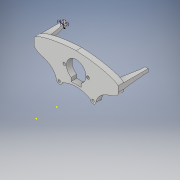
# Autodesk Inventor part: turret_base
Saved by Autodesk Inventor 2019 (Build 230136000, 136)
## iProperties
Created: 2019-04-21
Part Number: turret_base
Material: Ogólny
Document SubType Name: Modeling
Designer: terg
Density: 1 g/cm^3
Appearance: Domyślna
Author: terg
Autodesk Inventor part; units mm, degrees
ref_plane "XZ Plane" through (0, 0, 0) normal (0, 1, 0) x (-1, 0, 0)
sketch "Szkic2" plane through (0, 0, 0) normal (0, 0, 1) x (1, 0, 0)
  line L0 (4.75, 102.75) -> (9.25, 102.75)
  line L1 (9.25, 102.75) -> (9.25, 107.25)
  line L2 (9.25, 107.25) -> (4.75, 107.25)
  line L3 (4.75, 107.25) -> (4.75, 102.75)
  line L4 (4.75, 102.75) -> (9.25, 107.25) construction
  line L5 (9.25, 102.75) -> (4.75, 107.25) construction
  point P0 (0, 0)
  point P1 (64.95, 71.5)
  point P2 (7, 105)
  dimension "d1" = 4.5
  dimension "d2" = 4.5
  constraints: 12 end point, 2 midpoint, 2 parallel, 1 horizontal, 1 perpendicular, 1 other
  measures "d1" distance of L2.end L1.end
  measures "d2" distance of L1.end L0.end
ref_plane "Płaszczyzna konstrukcyjna1" through (64.95, 71.5, 0) normal (1, 0, 0) x (0, 1, 0)
ref_plane "Płaszczyzna konstrukcyjna2" through (0, 0, 29) normal (0, 0, 1) x (1, 0, 0)
sketch "Szkic3" plane through (0, 0, 29) normal (0, 0, 1) x (1, 0, 0)
  circle A0 centre (40.75, 71) radius 1.75 projected
  point P0 (0, 0)
extrude "Wyciągnięcie proste1" add sketch "Szkic2" against normal blind 6
sketch "Szkic4" plane through (0, 0, 0) normal (0, 0, 1) x (1, 0, 0)
  line L0 (4.75, 102.75) -> (9.25, 102.75) projected
  line L1 (9.25, 102.75) -> (9.25, 107.25) projected
  line L2 (9.25, 107.25) -> (4.75, 107.25) projected
  line L3 (4.75, 107.25) -> (4.75, 102.75) projected
  point P0 (0, 0)
sketch "Szkic5" plane through (0, 0, 29) normal (0, 0, 1) x (1, 0, 0)
  line L0 (64.95, 149.0685) -> (64.95, -24.8448) construction
  line L1 (64.95, 88) -> (64.95, 96) construction
  line L2 (64.95, 96) -> (47.95, 96) construction
  circle A0 centre (47.95, 96) radius 2
  line L3 (64.95, 96) -> (64.95, 84) construction
  line L4 (64.95, 84) -> (57.7389, 84) construction
  arc A1 (64.95, 110) -> (57.7389, 84) centre (64.95, 96) ccw
  line L5 (57.7389, 84) -> (57.7389, 79)
  line L6 (57.7389, 79) -> (64.95, 79)
  circle A2 centre (40.75, 71) radius 1.75 projected
  line L7 (64.95, 96) -> (81.95, 96) construction
  circle A3 centre (81.95, 96) radius 2
  line L8 (64.95, 84) -> (72.1611, 84) construction
  arc A4 (72.1611, 84) -> (64.95, 110) centre (64.95, 96) ccw
  line L9 (72.1611, 84) -> (72.1611, 79)
  line L10 (72.1611, 79) -> (64.95, 79)
  circle A5 centre (89.15, 71) radius 1.75
  arc A6 (36.75, 71) -> (44.75, 71) centre (40.75, 71) ccw
  arc A7 (85.15, 71) -> (93.15, 71) centre (89.15, 71) ccw
  arc A8 (85.15, 71) -> (44.75, 71) centre (64.95, 34.5448) ccw
  spline S0 degree 3 poles (4.75, 99.25) (3.3447, 87.1152) (30.6878, 94.0489) (36.75, 71) knots 0 0 0 0 1 1 1 1
  spline S1 degree 3 poles (125.15, 99.25) (126.5553, 87.1152) (99.2122, 94.0489) (93.15, 71) knots 0 0 0 0 1 1 1 1
  spline S2 degree 4 poles (4.75, 107.25) (7.6598, 112.7952) (35.9373, 119.5714) (52.5371, 120.1837) (64.95, 120.886) knots 0 0 0 0 0 1 1 1 1 1
  spline S3 degree 4 poles (125.15, 107.25) (122.2402, 112.7952) (93.9627, 119.5714) (77.3629, 120.1837) (64.95, 120.886) knots 0 0 0 0 0 1 1 1 1 1
  line L11 (125.15, 107.25) -> (125.15, 99.25)
  line L12 (4.75, 107.25) -> (4.75, 99.25)
  point P0 (0, 0)
  point P1 (50.95, 96)
  point P2 (78.95, 96)
  point P3 (7.7703, 93.2829)
  point P4 (21.1067, 88)
  point P5 (122.1297, 93.2829)
  point P6 (108.7933, 88)
  point P7 (10.3549, 111.0646)
  point P8 (29.8942, 116.7506)
  point P9 (51.4593, 119.9555)
  point P10 (119.5451, 111.0646)
  point P11 (100.0058, 116.7506)
  point P12 (78.4407, 119.9555)
  dimension "d7" = 17
  dimension "d8" = 4
  dimension "d9" = 12
  dimension "d10" = 5
  dimension "d13" = 4
  dimension "d14" = 8
  constraints: 24 end point, 18 symmetric about line, 14 point on circle, 8 centre point, 7 coincident, 5 point on line, 3 vertical, 2 perpendicular, 1 horizontal, 23 other
  measures "d7" distance of L2.start L2.end
  measures "d8" diameter of A0
  measures "d9" distance of L3.start L3.end
  measures "d10" distance of L5.start L5.end
  measures "d13" distance of A2.centre A6.start
  measures "d14" distance of A6.start A6.end
extrude "Wyciągnięcie proste2" add sketch "Szkic5" along normal blind 8
sketch "Szkic6" plane through (0, 0, 29) normal (0, 0, -1) x (-1, 0, 0)
  line L0 (-9.25, 107.25) -> (-4.75, 107.25) projected
  line L1 (-4.75, 107.25) -> (-4.75, 99.25) projected
  line L2 (-4.75, 107.25) -> (-14.75, 107.25)
  line L3 (-14.75, 107.25) -> (-14.75, 99.25)
  line L4 (-14.75, 99.25) -> (-4.75, 99.25)
  line L5 (-4.75, 99.25) -> (-4.75, 107.25)
  line L6 (-64.95, -24.1772) -> (-64.95, 145.0632) construction
  point P0 (0, 0)
  point P1 (-125.15, 107.25)
  dimension "d19" = 10
  dimension "d20" = 8
  constraints: 8 end point, 2 parallel, 1 horizontal, 1 perpendicular, 1 symmetric about line
  measures "d19" distance of L4.end L3.end
  measures "d20" distance of L3.end L2.end
sketch "Szkic7" plane through (0, 0, 0) normal (0, 0, 1) x (1, 0, 0)
  line L0 (4.75, 102.75) -> (9.25, 102.75) projected
  line L1 (9.25, 102.75) -> (9.25, 107.25) projected
  line L2 (9.25, 107.25) -> (4.75, 107.25) projected
  line L3 (4.75, 107.25) -> (4.75, 102.75) projected
  line L4 (4.75, 102.75) -> (9.25, 102.75) projected
  line L5 (4.75, 102.75) -> (9.25, 102.75)
  line L6 (9.25, 102.75) -> (9.25, 107.25)
  line L7 (9.25, 107.25) -> (4.75, 107.25)
  line L8 (4.75, 107.25) -> (4.75, 102.75)
  point P0 (0, 0)
  dimension "d21" = 4.5
  dimension "d22" = 4.5
  constraints: 8 end point, 2 parallel, 1 horizontal, 1 perpendicular
  measures "d21" distance of L7.end L1.end
  measures "d22" distance of L1.end L5.end
loft "Wyciągnięcie złożone1" add profiles "Szkic6" section 1 edges at (7, 102.75, 0) (9.25, 105, 0) (7, 107.25, 0) (4.75, 105, 0)
mirror "Odbij1" about plane through (64.95, 71.5, 0) normal (1, 0, 0) of "Wyciągnięcie złożone1", "Wyciągnięcie proste1"
